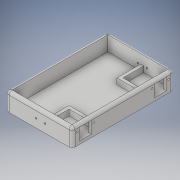
# Autodesk Inventor part: P1794_001_basManette
Saved by Autodesk Inventor 2019 (Build 230136000, 136)
## iProperties
Created: 2019-04-29
Part Number: P1794_001_basManette
Material: Générique
Document SubType Name: Modeling
Designer: Joan.MAILLARD
Density: 1 g/cm^3
Appearance: Par défaut
Author: Joan.MAILLARD
Autodesk Inventor part; units mm, degrees
ref_plane "YZ Plane" through (0, 0, 0) normal (1, 0, 0) x (0, 1, 0)
ref_plane "XZ Plane" through (0, 0, 0) normal (0, 1, 0) x (-1, 0, 0)
ref_plane "XY Plane" through (0, 0, 0) normal (0, 0, 1) x (1, 0, 0)
sketch "Esquisse1" plane through (0, 0, 0) normal (0, 1, 0) x (-1, 0, 0)
  line L0 (-55, 85) -> (55, 85)
  line L1 (55, 85) -> (55, -85)
  line L2 (55, -85) -> (-55, -85)
  line L3 (-55, -85) -> (-55, 85)
  line L4 (-55, 85) -> (55, -85) construction
  line L5 (55, 85) -> (-55, -85) construction
  point P0 (0, 0)
  dimension "d0" = 170
  dimension "d1" = 110
  constraints: 12 end point, 2 midpoint, 2 parallel, 1 horizontal, 1 perpendicular
  measures "d0" distance of L0.end L1.end
  measures "d1" distance of L1.end L2.end
extrude "Extrusion1" add sketch "Esquisse1" along normal blind 30
fillet "Congé1" radius 5 4 edges at (0, 30, 85) (55, 30, 0) (0, 30, -85) (-55, 30, 0)
fillet "Congé2" radius 5 8 edges at (-53.5355, 28.5355, -83.5355) (-55, 12.5, -85) (-53.5355, 28.5355, 83.5355) (-55, 12.5, 85) (53.5355, 28.5355, -83.5355) (55, 12.5, -85) (53.5355, 28.5355, 83.5355) (55, 12.5, 85)
sketch "Esquisse2" plane through (0, 30, 0) normal (0, 1, 0) x (1, 0, 0)
  line L0 (-50, -80) -> (-50, 80) projected
  line L1 (-50, 80) -> (50, 80) projected
  line L2 (-50, -80) -> (50, -80)
  line L3 (50, -80) -> (50, 80)
  line L4 (50, 80) -> (-50, 80)
  line L5 (-50, 80) -> (-50, -80)
  point P0 (0, 0)
  constraints: 8 end point, 2 parallel, 1 horizontal, 1 perpendicular
extrude "Extrusion2" cut sketch "Esquisse2" against normal blind 25
sketch "Esquisse3" plane through (55, 0, -85) normal (0, 0, -1) x (-1, 0, 0)
  line L0 (55, 14) -> (40, 14) construction
  line L1 (105, 0) -> (0, 0) construction
  line L2 (0, 0) -> (0, 25) construction
  point P0 (55, 0)
  dimension "d15" = 14
  dimension "d16" = 15
  dimension "d17" = 40
  constraints: 2 end point, 1 horizontal
  measures "d15" distance between parallel lines of L1 L0
  measures "d16" distance of L0.end L0.start
  measures "d17" distance from line of L2 L0.end
hole "Perçage1" at (15, 14, -85) at (0, 14, -85) direction (0, 0, 1) diameter 2.459 depth 8.8 tip angle 118 thread size "M3x0.5" class "6H" standard "ISO Metric profile"
sketch "Esquisse4" plane through (-50, 0, 85) normal (0, 0, 1) x (1, 0, 0)
  line L0 (45, 14) -> (60, 14) construction
  line L1 (100, 25) -> (100, 0) construction
  line L2 (100, 0) -> (0, 0) construction
  point P0 (50, 0)
  dimension "d25" = 15
  dimension "d26" = 40
  dimension "d27" = 14
  constraints: 2 end point, 1 horizontal
  measures "d25" distance of L0.start L0.end
  measures "d26" distance from line of L1 L0.end
  measures "d27" distance between parallel lines of L2 L0
hole "Perçage2" at (-5, 14, 85) at (10, 14, 85) direction (0, 0, -1) diameter 2.459 depth 8.8 tip angle 118 thread size "M3x0.5" class "6H" standard "ISO Metric profile"
sketch "Esquisse5" plane through (55, 0, 80) normal (1, 0, 0) x (0, 0, -1)
  line L0 (160, 25) -> (0, 25) projected
  line L1 (0, 5) -> (160, 5) projected
  line L2 (7.5, 25) -> (27.5, 25)
  line L3 (27.5, 25) -> (27.5, 5)
  line L4 (27.5, 5) -> (7.5, 5)
  line L5 (7.5, 5) -> (7.5, 25)
  line L6 (0, 0) -> (0, 25) projected
  line L7 (152.5, 25) -> (132.5, 25)
  line L8 (132.5, 25) -> (132.5, 5)
  line L9 (132.5, 5) -> (152.5, 5)
  line L10 (152.5, 5) -> (152.5, 25)
  line L11 (160, 25) -> (160, 0) projected
  point P0 (80, 0)
  dimension "d40" = 7.5
  dimension "d41" = 20
  dimension "d42" = 7.5
  dimension "d43" = 20
  constraints: 16 end point, 4 parallel, 4 point on line, 2 horizontal, 2 perpendicular
  measures "d40" distance between parallel lines of L6 L5
  measures "d41" distance between parallel lines of L3 L5
  measures "d42" distance between parallel lines of L11 L10
  measures "d43" distance between parallel lines of L10 L8
extrude "Extrusion3" cut sketch "Esquisse5" against normal blind 5 contours L10 L1 L8 L0 | L3 L1 L5 L0
sketch "Esquisse6" plane through (0, 5, 0) normal (0, 1, 0) x (1, 0, 0)
  line L0 (-50, 80) -> (50, 80) projected
  line L1 (50, -80) -> (-50, -80) projected
  line L2 (25, -80) -> (30, -80)
  line L3 (50, 52.5) -> (50, -52.5) projected
  line L4 (50, 45) -> (10, 45)
  line L5 (10, 45) -> (10, 40)
  line L6 (10, 40) -> (50, 40)
  line L7 (50, 40) -> (50, 45)
  line L8 (10, 40) -> (5, 40)
  line L9 (5, 40) -> (5, 80)
  line L10 (5, 80) -> (10, 80)
  line L11 (10, 80) -> (10, 40)
  line L12 (55, 52.5) -> (50, 52.5) projected
  line L13 (50, 80) -> (50, -80) projected
  line L14 (10, -80) -> (5, -80)
  line L15 (5, -80) -> (5, -40)
  line L16 (5, -40) -> (10, -40)
  line L17 (10, -40) -> (10, -80)
  line L18 (50, -40) -> (10, -40)
  line L19 (10, -40) -> (10, -45)
  line L20 (10, -45) -> (50, -45)
  line L21 (50, -45) -> (50, -40)
  point P0 (0, 0)
  point P1 (7.5, -40)
  dimension "d44" = 5
  dimension "d45" = 5
  dimension "d46" = 7.5
  dimension "d47" = 40
  dimension "d48" = 5
  dimension "d49" = 7.5
  dimension "d50" = 5
  dimension "d51" = 40
  constraints: 34 end point, 8 parallel, 7 point on line, 4 horizontal, 4 perpendicular, 1 midpoint
  measures "d44" distance between parallel lines of L6 L4
  measures "d45" distance between parallel lines of L9 L11
  measures "d46" distance between parallel lines of L4 L12
  measures "d47" distance between parallel lines of L13 L11
  measures "d48" distance between parallel lines of L20 L18
  measures "d49" distance from line of L20 L3.end
  measures "d50" distance between parallel lines of L17 L15
  measures "d51" distance between parallel lines of L17 L13
extrude "Extrusion4" add sketch "Esquisse6" along normal blind 10 contours L0 L11 L5 L8 L9 | L4 L3 L6 L5 | L20 L17 L18 L3 | L1 L15 L16 L17
sketch "Esquisse8" plane through (55, 0, 80) normal (1, 0, 0) x (0, 0, -1)
  line L0 (0, 25) -> (0, 0) construction
  line L1 (0, 20) -> (3.75, 20) construction
  line L2 (3.75, 20) -> (7.5, 20) construction
  line L3 (7.5, 25) -> (7.5, 5) construction
  line L4 (3.75, 20) -> (3.75, 15) construction
  line L5 (0, 15) -> (35, 15) construction
  line L6 (3.75, 20) -> (3.75, 25) construction
  line L7 (160, 25) -> (0, 25) construction
  line L8 (31.25, 20) -> (31.25, 25) construction
  line L9 (31.25, 20) -> (27.5, 20) construction
  line L10 (27.5, 5) -> (27.5, 25) construction
  line L11 (128.75, 20) -> (128.75, 25) construction
  line L12 (128.75, 20) -> (132.5, 20) construction
  line L13 (156.25, 20) -> (156.25, 25) construction
  line L14 (156.25, 20) -> (152.5, 20) construction
  line L15 (152.5, 25) -> (152.5, 5) construction
  line L16 (132.5, 5) -> (132.5, 25) construction
  point P0 (80, 0)
  constraints: 20 end point, 8 equal length, 8 point on line, 3 perpendicular, 3 vertical, 2 horizontal, 1 parallel, 5 other
hole "Perçage4" at (55, 20, 76.25) at (55, 20, 48.75) at (55, 20, -48.75) at (55, 20, -76.25) direction (-1, 0, 0) diameter 3 depth 8.8 tip angle 118
equation "\"d45\" = d44"
equation "\"d50\" = d45"
equation "\"d51\" = d47"
